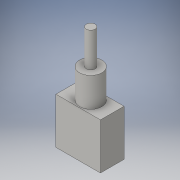
# Autodesk Inventor part: RTS Switch
Saved by Autodesk Inventor 2016 (Build 200138000, 138)
## iProperties
Created: 2016-10-07
Part Number: RTS Switch
Material: Generic
Document SubType Name: Modeling
Designer: sullir
Density: 1 g/cm^3
Appearance: Default
Author: sullir
Autodesk Inventor part; units mm, degrees
ref_plane "YZ Plane" through (0, 0, 0) normal (1, 0, 0) x (0, 1, 0)
ref_plane "XZ Plane" through (0, 0, 0) normal (0, 1, 0) x (-1, 0, 0)
ref_plane "XY Plane" through (0, 0, 0) normal (0, 0, 1) x (1, 0, 0)
sketch "Sketch1" plane through (0, 0, 0) normal (0, 0, 1) x (1, 0, 0)
  line L0 (-1.2233, 5.2741) -> (11.6799, 5.2741)
  line L1 (11.6799, 5.2741) -> (11.6799, -8.0863)
  line L2 (11.6799, -8.0863) -> (-1.2233, -8.0863)
  line L3 (-1.2233, -8.0863) -> (-1.2233, 5.2741)
  point P0 (0, 0)
  dimension "d0" = 12.9032
  dimension "d1" = 13.3604
  constraints: 8 end point, 2 parallel, 1 horizontal, 1 perpendicular
  measures "d0" distance of L0.start L0.end
  measures "d1" distance of L0.end L1.end
extrude "Extrusion1" add sketch "Sketch1" along normal blind 6.858
sketch "Sketch2" plane through (-1.2233, 5.2741, 0) normal (0, 1, 0) x (1, 0, 0)
  circle A0 centre (6.5644, -3.3352) radius 3.2291
  line L0 (12.9032, 0) -> (12.9032, -6.858) projected
  point P0 (1.2233, 0)
  dimension "d4" = 6.3388
  constraints: 1 centre point
  measures "d4" distance from line of L0 A0.centre
extrude "Extrusion2" add sketch "Sketch2" along normal blind 8.509
sketch "Sketch3" plane through (5.3411, 13.7831, 3.3352) normal (0, 1, 0) x (1, 0, 0)
  circle A0 centre (0, 0) radius 1.2757
  point P0 (-5.3411, 3.3352)
  constraints: 1 centre point
extrude "Extrusion3" add sketch "Sketch3" along normal blind 9.9822
body "Solid1"
